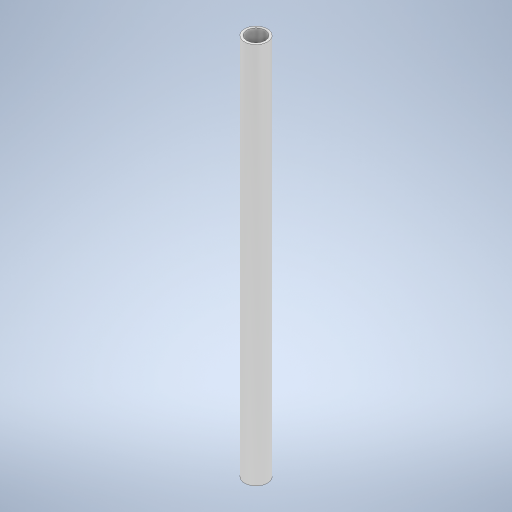
# Autodesk Inventor part: InsertTube
Saved by Autodesk Inventor 2024 (Build 280153000, 153)
## iProperties
Created: 2023-09-24
Part Number: InsertTube
Material: Stainless Steel AISI 304
Document SubType Name: Modeling
Designer: schanen
Density: 8 g/cm^3
Appearance: Chrome - Satin
Author: schanen
Autodesk Inventor part; units mm, degrees
ref_plane "YZ Plane" through (0, 0, 0) normal (1, 0, 0) x (0, 1, 0)
ref_plane "XZ Plane" through (0, 0, 0) normal (0, 1, 0) x (-1, 0, 0)
ref_plane "XY Plane" through (0, 0, 0) normal (0, 0, 1) x (1, 0, 0)
sketch "Sketch1" plane through (0, 0, 0) normal (0, 0, 1) x (1, 0, 0)
  line L0 (-2.4, 0) -> (-3, 0)
  line L1 (-3, 0) -> (-3, 100)
  line L2 (-3, 100) -> (-2.4, 100)
  line L3 (-2.4, 100) -> (-2.4, 0)
  line L4 (0, -20) -> (0, 120) projected
  point P0 (0, 0)
  dimension "d0" = 3
  dimension "d1" = 0.6
  dimension "d2" = 100
  constraints: 8 end point, 2 parallel, 1 horizontal, 1 perpendicular
  measures "d0" distance from line of point (0, 0) L1
  measures "d1" distance between parallel lines of L1 L3
  measures "d2" distance of L0.end L1.end
revolve "Revolution1" add sketch "Sketch1" angle 360 about axis through (0, -10, 0) along (0, 1, 0)
body "Solid1"
